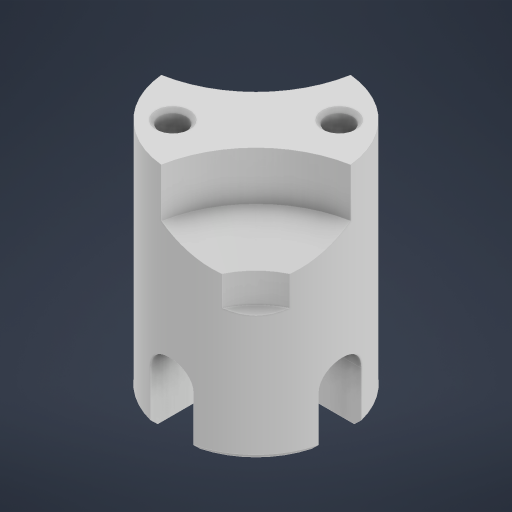
# Autodesk Inventor part: mount-stem
Saved by Autodesk Inventor 2024 (Build 280153000, 153)
## iProperties
Created: 2024-05-22
Part Number: mount-stem
Material: Generic
Document SubType Name: Modeling
Designer: loren
Density: 1 g/cm^3
Appearance: Default
Author: loren
## iProperties of the stored document mount-stem_3DPrint.ipt
Created: 2026-02-06
Part Number: mount-stem_3DPrint
Material: Generic
Document SubType Name: Modeling
Designer: lokies
Density: 1 g/cm^3
Appearance: Default
Author: lokies
Autodesk Inventor part; units mm, degrees
ref_plane "XZ Plane" through (0, 0, 0) normal (0, 1, 0) x (-1, 0, 0)
sketch "Sketch1" plane through (0, 0, 0) normal (0, 1, 0) x (-1, 0, 0)
  circle A0 centre (0, 0) radius 12.5
  dimension "d0" = 25
  constraints: 1 centre point, 1 coincident
  measures "d0" diameter of A0
extrude "Extrusion1" add sketch "Sketch1" along normal blind 19 and the other way blind 15
sketch "Sketch2" plane through (0, 0, 0) normal (0, 0, 1) x (1, 0, 0)
  line L0 (-5.25, -15) -> (-5.25, -7.5)
  arc A0 (5.25, -7.5) -> (-5.25, -7.5) centre (0, -7.5) ccw
  line L1 (5.25, -7.5) -> (5.25, -15)
  line L2 (5.25, -15) -> (-5.25, -15)
  line L3 (-3.1, -15) -> (-3.1, -7.5)
  arc A1 (3.1, -7.5) -> (-3.1, -7.5) centre (0, -7.5) ccw
  line L4 (3.1, -7.5) -> (3.1, -15)
  line L5 (0, 0) -> (0, -15) construction
  line L6 (-12.5, -15) -> (12.5, -15) projected
  point P0 (0, -7.5)
  dimension "d5" = 10.5
  dimension "d6" = 6.2
  constraints: 12 end point, 4 point on circle, 4 tangent, 3 point on line, 2 centre point, 2 midpoint, 2 perpendicular, 2 vertical, 1 coincident, 1 concentric, 1 parallel
  measures "d5" distance between parallel lines of L1 L0
  measures "d6" distance between parallel lines of L4 L3
extrude "Extrusion2" cut sketch "Sketch2" along normal mid plane 10.5
extrude "Extrusion3" cut sketch "Sketch2" against normal through all both and the other way through all contours L3 A1 L4 L2
pattern_circular "Circular Pattern1" count 2 over 90 about axis through (0, -10, 0) along (0, 1, 0) of "Extrusion2", "Extrusion3"
ref_plane "Work Plane2" through (0, 0, 0) normal (0.7071, 0, -0.7071) x (0, 1, 0)
sketch "Sketch5" plane through (0, 0, 0) normal (0.7071, 0, -0.7071) x (0, 1, 0)
  line L0 (19, -21.9203) -> (-2.0622, -21.9203)
  line L1 (-21.8122, 0) -> (25.8729, 0) projected
  line L2 (19, -12.5) -> (19, 12.5) projected
  line L3 (19, -21.9203) -> (19, -4.9203)
  line L4 (19, -4.9203) -> (12, -4.9203)
  line L5 (12, -4.9203) -> (8.2472, -11.4203)
  line L6 (8.2472, -11.4203) -> (4, -11.4203)
  line L7 (4, -11.4203) -> (-2.0622, -21.9203)
  point P0 (0, 0)
  dimension "d40" = 21.9203
  dimension "d41" = 34
  dimension "d42" = 7
  dimension "d43" = 21
  dimension "d44" = 15
  dimension "d45" = 60
  constraints: 12 end point, 3 horizontal, 1 parallel, 1 point on line, 1 vertical
  measures "d40" distance between parallel lines of L0 L1
  measures "d41" diameter of L4 L0
  measures "d42" distance of L3.end L4.end
  measures "d43" diameter of L6 L0
  measures "d44" distance from line of L6.end L3
  measures "d45" angle of L4 L5
revolve "Revolution1" cut sketch "Sketch5" angle 360 about axis through (-15.5, 19, -15.5) along (0, -1, 0)
sketch "Sketch6" plane through (0, 19, 0) normal (0, 1, 0) x (1, 0, 0)
  circle A0 centre (6, 6) radius 1.9
  point P0 (0, 0)
  dimension "d47" = 3.8
  dimension "d48" = 6
  dimension "d49" = 6
  constraints: 1 centre point
  measures "d47" diameter of A0
  measures "d48" horizontal distance of A0.centre point (0, 0)
  measures "d49" horizontal distance of A0.centre point (0, 0)
extrude "Extrusion9" cut sketch "Sketch6" against normal blind 20
chamfer "Chamfer2" distance 0.5 angle 45 1 edges at (4.1, 19, -6)
pattern_circular "Circular Pattern4" count 2 over 360 about axis through (0, -10, 0) along (0, 1, 0) of "Revolution1", "Extrusion9", "Chamfer2"
chamfer "Chamfer1" distance 1 angle 45 4 edges at (8.8388, -15, 8.8388) (-8.8388, -15, 8.8388) (-8.8388, -15, -8.8388) (8.8388, -15, -8.8388)
equation "\"d49\" = d48"
body "Solid1"
